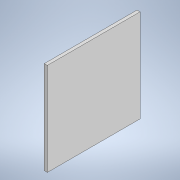
# Autodesk Inventor part: front
Saved by Autodesk Inventor 2021 (Build 250183000, 183)
## iProperties
Created: 2021-07-08
Part Number: front
Material: Generic
Document SubType Name: Modeling
Designer: almas
Density: 1 g/cm^3
Appearance: Default
Author: almas
Autodesk Inventor part; units mm, degrees
ref_plane "YZ Plane" through (0, 0, 0) normal (1, 0, 0) x (0, 1, 0)
ref_plane "XZ Plane" through (0, 0, 0) normal (0, 1, 0) x (-1, 0, 0)
ref_plane "XY Plane" through (0, 0, 0) normal (0, 0, 1) x (1, 0, 0)
sketch "Sketch1" plane through (0, 0, 0) normal (1, 0, 0) x (0, 1, 0)
  line L0 (0, 0) -> (381, 0)
  line L1 (381, 0) -> (381, -381)
  line L2 (381, -381) -> (0, -381)
  line L3 (0, -381) -> (0, 0)
  dimension "d0" = 381
  dimension "d1" = 381
  constraints: 8 end point, 2 parallel, 1 horizontal, 1 perpendicular
  measures "d0" distance of L0.end L1.end
  measures "d1" distance of L1.end L2.end
extrude "Extrusion1" add sketch "Sketch1" along normal blind 12.7
sketch "Sketch2" plane through (0, 0, 0) normal (-1, 0, 0) x (0, 0, 1)
  line L0 (-355.6, 355.6) -> (-25.4, 355.6)
  line L1 (-25.4, 355.6) -> (-25.4, 25.4)
  line L2 (-25.4, 25.4) -> (-355.6, 25.4)
  line L3 (-355.6, 25.4) -> (-355.6, 355.6)
  line L4 (-381, 0) -> (-381, 381) projected
  line L5 (0, 381) -> (0, 0) projected
  line L6 (0, 0) -> (-381, 0) projected
  line L7 (-381, 381) -> (0, 381) projected
  dimension "d4" = 25.4
  dimension "d5" = 25.4
  dimension "d6" = 25.4
  dimension "d7" = 25.4
  constraints: 8 end point, 2 parallel, 1 horizontal, 1 perpendicular
  measures "d4" distance between parallel lines of L4 L3
  measures "d5" distance between parallel lines of L5 L1
  measures "d6" distance between parallel lines of L6 L2
  measures "d7" distance between parallel lines of L7 L0
extrude "Extrusion2" add sketch "Sketch2" along normal blind 12.7 contours L0 L1 L2 L3
sketch "Sketch3" plane through (-12.7, 0, 0) normal (-1, 0, 0) x (0, 0, 1)
  line L0 (-330.2, 76.2) -> (-279.4, 76.2)
  line L1 (-279.4, 76.2) -> (-279.4, 50.8)
  line L2 (-279.4, 50.8) -> (-330.2, 50.8)
  line L3 (-330.2, 50.8) -> (-330.2, 76.2)
  line L4 (-355.6, 355.6) -> (-355.6, 25.4) projected
  line L5 (-355.6, 25.4) -> (-25.4, 25.4) projected
  point P0 (0, 0)
  dimension "d10" = 25.4
  dimension "d11" = 25.4
  dimension "d12" = 25.4
  dimension "d13" = 50.8
  constraints: 8 end point, 2 parallel, 1 horizontal, 1 perpendicular
  measures "d10" distance between parallel lines of L4 L3
  measures "d11" distance between parallel lines of L5 L2
  measures "d12" distance of L0.end L1.end
  measures "d13" distance of L0.start L0.end
extrude "Extrusion3" add sketch "Sketch3" along normal blind 5.08
sketch "Sketch4" plane through (-12.7, 0, 0) normal (-1, 0, 0) x (0, 0, 1)
  line L0 (-101.6, 76.2) -> (-50.8, 76.2)
  line L1 (-50.8, 76.2) -> (-50.8, 50.8)
  line L2 (-50.8, 50.8) -> (-101.6, 50.8)
  line L3 (-101.6, 50.8) -> (-101.6, 76.2)
  line L4 (-25.4, 25.4) -> (-25.4, 355.6) projected
  line L5 (-355.6, 25.4) -> (-25.4, 25.4) projected
  point P0 (0, 0)
  dimension "d16" = 25.4
  dimension "d17" = 25.4
  dimension "d18" = 25.4
  dimension "d19" = 50.8
  constraints: 8 end point, 2 parallel, 1 horizontal, 1 perpendicular
  measures "d16" distance between parallel lines of L4 L1
  measures "d17" distance between parallel lines of L5 L2
  measures "d18" distance of L2.end L0.start
  measures "d19" distance of L0.start L0.end
extrude "Extrusion4" add sketch "Sketch4" along normal blind 5.08
sketch "Sketch5" plane through (-17.78, 0, 0) normal (-1, 0, 0) x (0, 0, 1)
  line L0 (-317.5, 69.85) -> (-292.1, 69.85)
  line L1 (-292.1, 69.85) -> (-292.1, 57.15)
  line L2 (-292.1, 57.15) -> (-317.5, 57.15)
  line L3 (-317.5, 57.15) -> (-317.5, 69.85)
  line L4 (-279.4, 50.8) -> (-279.4, 76.2) projected
  line L5 (-330.2, 76.2) -> (-330.2, 50.8) projected
  line L6 (-279.4, 76.2) -> (-330.2, 76.2) projected
  line L7 (-330.2, 50.8) -> (-279.4, 50.8) projected
  point P0 (0, 0)
  dimension "d22" = 12.7
  dimension "d23" = 12.7
  dimension "d24" = 6.35
  dimension "d25" = 6.35
  constraints: 8 end point, 2 parallel, 1 horizontal, 1 perpendicular
  measures "d22" distance between parallel lines of L4 L1
  measures "d23" distance between parallel lines of L5 L3
  measures "d24" distance between parallel lines of L6 L0
  measures "d25" distance between parallel lines of L7 L2
extrude "Extrusion5" cut sketch "Sketch5" against normal blind 5.08 contours L0 L1 L2 L3
sketch "Sketch6" plane through (-17.78, 0, 0) normal (-1, 0, 0) x (0, 0, 1)
  line L0 (-88.9, 69.85) -> (-63.5, 69.85)
  line L1 (-63.5, 69.85) -> (-63.5, 57.15)
  line L2 (-63.5, 57.15) -> (-88.9, 57.15)
  line L3 (-88.9, 57.15) -> (-88.9, 69.85)
  line L4 (-101.6, 76.2) -> (-101.6, 50.8) projected
  line L5 (-50.8, 50.8) -> (-50.8, 76.2) projected
  line L6 (-50.8, 76.2) -> (-101.6, 76.2) projected
  line L7 (-101.6, 50.8) -> (-50.8, 50.8) projected
  point P0 (0, 0)
  dimension "d28" = 12.7
  dimension "d29" = 12.7
  dimension "d30" = 6.35
  dimension "d31" = 6.35
  constraints: 8 end point, 2 parallel, 1 horizontal, 1 perpendicular
  measures "d28" distance between parallel lines of L4 L3
  measures "d29" distance between parallel lines of L5 L1
  measures "d30" distance between parallel lines of L6 L0
  measures "d31" distance between parallel lines of L7 L2
extrude "Extrusion6" cut sketch "Sketch6" against normal blind 5.08 contours L0 L1 L2 L3
body "Solid1"
